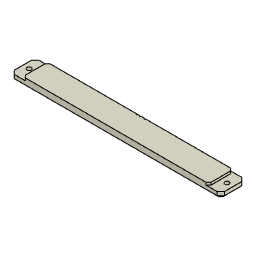
Front Panel - Template (Autodesk Fusion 360 design; units mm, degrees)
Autodesk Fusion 360 part; units mm, degrees
ref_plane "WorkPlane1" through (0, -117.8, 0) normal (0, 1, 0) x (0, 0, 1)
sketch "Sketch1" plane through (0, -117.8, 0) normal (0, 1, 0) x (1, 0, 0)
  line L0 (-88.4655, -26.8517) -> (89.2, -26.8517)
  line L1 (89.2, -26.8517) -> (89.2, 0)
  line L2 (89.2, 0) -> (-88.4655, 0)
  line L3 (-88.4655, 0) -> (-88.4655, -26.8517)
ref_plane "WorkPlane2" through (0, -123, 0) normal (0, 1, 0) x (0, 0, 1)
sketch "Sketch2" plane through (0, -123, 0) normal (0, 1, 0) x (1, 0, 0)
  line L0 (-88.4862, 0.0071) -> (88.5, 0.0071) construction
  line L1 (88.5, 0.0071) -> (88.5, -28.9292)
  line L2 (88.5, -28.9292) -> (87.9405, -29.5447) construction
  line L3 (-88.4655, 0) -> (-88.4655, -26.8517) construction
  line L4 (-88.4862, -26.8517) -> (89.2, -26.8517) construction
  line L5 (89.2, -26.8517) -> (89.2, 0) construction
  line L6 (88.5, -26.8517) -> (88.5, 0.0071)
  line L7 (-88.4862, -26.8517) -> (88.5, -26.8517)
  line L8 (88.5, 0.0071) -> (-88.4862, 0.0071)
  line L9 (-88.4862, -26.8517) -> (-88.4862, 0.0071)
  line L10 (85.5, -21.8517) -> (85.5, -7.8517)
  line L11 (-82.4864, -24.8517) -> (82.5, -24.8517)
  line L12 (82.5, -4.8517) -> (-82.4864, -4.8517)
  line L13 (-88.4655, -4.8517) -> (-88.5, -4.8517)
  line L14 (-85.4864, -21.8517) -> (-85.4864, -7.8517)
  line L15 (-85.4864, 0.0071) -> (-85.4864, 0.0039)
  line L16 (-75.4864, -24.8517) -> (-75.4864, -4.8517)
  line L17 (75.5, -24.8517) -> (75.5, -4.8517)
  line L18 (-75.4864, -4.8517) -> (-80.4972, -4.8517)
  line L19 (-85.4864, -24.8517) -> (-75.4864, -24.8517) construction
  line L20 (-80.4864, -24.8517) -> (-80.4972, -4.8517) construction
  line L21 (0.0068, -24.8517) -> (0.0068, -4.8517) construction
  arc A0 (-82.4864, -4.8517) -> (-85.4864, -7.8517) centre (-82.4864, -7.8517) ccw construction
  arc A1 (-85.4864, -21.8517) -> (-82.4864, -24.8517) centre (-82.4864, -21.8517) ccw construction
  arc A2 (85.5, -7.8517) -> (82.5, -4.8517) centre (82.5, -7.8517) ccw construction
  arc A3 (82.5, -24.8517) -> (85.5, -21.8517) centre (82.5, -21.8517) ccw construction
  circle A4 centre (-80.4836, -14.7936) radius 1.8
  circle A5 centre (80.4971, -14.7936) radius 1.8
  line L22 (-85.4864, -21.8517) -> (-82.4864, -24.8517)
  line L23 (-85.4864, -7.8517) -> (-82.4864, -4.8517)
  line L24 (85.5, -7.8517) -> (82.5, -4.8517)
  line L25 (85.5, -21.8517) -> (82.4977, -24.8517)
  point P0 (85.5, -4.8517)
  point P1 (85.5, -24.8517)
  dimension "d919" = 2
  dimension "d922" = 20
  dimension "d925" = 10
  dimension "d926" = 10
  dimension "d928" = 3
  dimension "d929" = 3
  dimension "d930" = 3
  dimension "d931" = 3
  dimension "d932" = 3.6
  constraint coincident L4 L6.start
  constraint coincident L1 L6.start
  constraint coincident L0.end L1.start
  constraint coincident L4.start L7.start
  constraint coincident L0.start L8.end
  constraint parallel L7 L11
  constraint parallel L9 L14
  constraint parallel L8 L12
  constraint coincident L3 L13.start
  constraint collinear L12 L13
  constraint coincident L0 L15.start
  constraint collinear L14 L15
  constraint parallel L6 L10
  constraint parallel L10 L17
  constraint coincident L11 L17.start
  constraint coincident L12 L17.end
  constraint parallel L14 L16
  constraint perpendicular L14 L18
  constraint perpendicular L16 L19
  constraint midpoint L19 L20.start
  constraint coincident L12 L21.end
  constraint tangent L12 A0
  constraint tangent L14 A0
  constraint coincident L11 L21.start
  constraint coincident L19.start L14
  constraint coincident L11 L19.start
  constraint tangent L14 A1
  constraint tangent L11 A1
  constraint coincident L12 P0
  constraint coincident L10 P0
  constraint tangent L12 A2
  constraint tangent L10 A2
  constraint coincident L11 P1
  constraint coincident L10 P1
  constraint tangent L11 A3
  constraint tangent L10 A3
  constraint symmetric L21 A4 A5
  constraint coincident L12 L16.end
  constraint coincident L11 L16.start
  constraint vertical L16
  constraint horizontal L12
  constraint vertical L10
  constraint symmetric L21 L12.end L12.start
  constraint symmetric L21 L14.end L10.end
  constraint symmetric L21 L14.start L10.start
  constraint coincident L11 L25.end
  constraint coincident L10 A3.end
  constraint coincident L10 A2.start
  measures "d919" distance of L7 L11
  measures "d922" distance of P0 P1
  measures "d925" distance of L10 L17
  measures "d926" distance of L14 L16
  measures "d928" radius of A0
  measures "d929" radius of A1
  measures "d930" radius of A2
  measures "d931" radius of A3
  measures "d932" diameter of A4
extrude "Extrude1" add sketch "Sketch2" along normal blind 4 contours L11 L12 L16 L17
extrude "Extrude2" add sketch "Sketch2" along normal blind 2 contours L10 L11 L12 L17 L24 L25 | L11 L12 L14 L16 L18 L22 L23
chamfer "Chamfer1" distance 2 angle 45 4 edges at (-75.4864, -120, 24.8517) (-75.4864, -120, 4.8517) (75.5, -120, 4.8517) (75.5, -120, 24.8517)
move_body "Move1" bodies 1 to x (1, 0, 0) y (0, 0, 1) z (0, -1, 0) at (0, -118.1483, 127.8517)
extrude "Extrude3" add 3 faces at (-25.1576, -129.6667, 4.8517) (-79.352, -140.2322, 4.8517) (79.3648, -140.2322, 4.8517) along direction (0, 0, -1) blind 3
chamfer "Chamfer2" distance 2 angle 45 8 edges at (85.5, -133, 1.8517) (83.9988, -141.5, 1.8517) (0.0056, -143, 1.8517) (-83.9864, -141.5, 1.8517) (-85.4864, -133, 1.8517) (-83.9864, -124.5, 1.8517) (0.0068, -123, 1.8517) (84, -124.5, 1.8517)
sketch "Sketch3" plane through (0, -123, 0) normal (0, 1, 0) x (-1, 0, 0)
  line L0 (-82.5, 3.8517) -> (82.4864, 3.8517)
  line L1 (82.4864, 3.8517) -> (82.4864, 6.8517)
  line L2 (82.4864, 6.8517) -> (73.4864, 6.8517)
  line L3 (73.4864, 6.8517) -> (73.4864, 8.8517)
  line L4 (73.4864, 8.8517) -> (-73.5, 8.8517)
  line L5 (-73.5, 8.8517) -> (-73.5, 6.8517)
  line L6 (-73.5, 6.8517) -> (-82.5, 6.8517)
  line L7 (-82.5, 6.8517) -> (-82.5, 3.8517)
  dimension "d11" = 5
  text T0 "V1" font "Arial" height 5 align centre spacing 1 along the path L0 letters at x, y, angle (-4.2786, 10.1751, 0) (0.3803, 10.1751, 0)
extrude "Extrude4" cut sketch "Sketch3" against normal blind 0.4 text T0
equation "d932 = large_m3"
equation "large_m3 = 3.6 mm"
